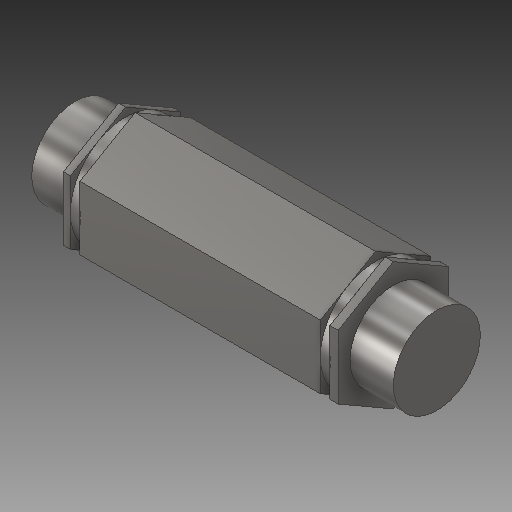
# Autodesk Inventor part: Hex Shaft 1
Saved by Autodesk Inventor 2019.4 (Build 234330000, 330)
## iProperties
Created: 2019-12-08
Part Number: Hex Shaft 1
Material: Steel, Mild
Document SubType Name: Modeling
Designer: admin
Density: 7.85 g/cm^3
Appearance: Semi-Polished
Mass: 40.5901 g
Surface Area: 20.2674 cm^2
Volume: 5.17072 cm^3
Author: admin
Autodesk Inventor part; units mm, degrees
ref_plane "YZ Plane" through (0, 0, 0) normal (1, 0, 0) x (0, 1, 0)
sketch "Sketch1" plane through (0, 0, 0) normal (0, 0, 1) x (1, 0, 0)
  line L0 (0, 0) -> (0, 5)
  line L1 (0, 5) -> (5, 5)
  line L2 (5, 5) -> (5, 8.4186)
  line L3 (5, 8.4186) -> (36.6, 8.4186)
  line L4 (36.6, 8.4186) -> (36.6, 5)
  line L5 (36.6, 5) -> (41.6, 5)
  line L6 (41.6, 5) -> (41.6, 0)
  line L7 (41.6, 0) -> (0, 0)
  dimension "d0" = 31.6
  dimension "d1" = 5
  dimension "d2" = 5
  dimension "d3" = 5
  constraints: 16 end point, 6 perpendicular, 2 point on line, 1 vertical
  measures "d0" distance of L2.end L3.end
  measures "d1" distance of L0.end L1.end
  measures "d2" distance of L4.end L5.end
  measures "d3" distance of L5.end L6.end
revolve "Revolution1" add sketch "Sketch1" angle 360 about axis through (41.6, 0, 0) along (-1, 0, 0)
sketch "Sketch2" plane through (36.6, 0, 0) normal (1, 0, 0) x (0, 0, -1)
  circle A0 centre (0, 0) radius 5 projected
  line L0 (0, 7.3323) -> (6.35, 3.6662)
  line L1 (6.35, 3.6662) -> (6.35, -3.6662)
  line L2 (6.35, -3.6662) -> (0, -7.3323)
  line L3 (0, -7.3323) -> (-6.35, -3.6662)
  line L4 (-6.35, -3.6662) -> (-6.35, 3.6662)
  line L5 (-6.35, 3.6662) -> (0, 7.3323)
  circle A1 centre (0, 0) radius 5 projected
  circle A2 centre (0, 0) radius 8.4186 projected
  dimension "d5" = 12.7
  constraints: 12 end point, 1 coincident, 13 other
  measures "d5" distance between parallel lines of L1 L4
extrude "Extrusion1" cut sketch "Sketch2" against normal up to surface (31.6 mm away) contours A2
ref_plane "Work Plane1" through (34.549, -3.6662, -6.35) normal (1, 0, 0) x (0, 0, -1)
sketch "Sketch3" plane through (34.549, -3.6662, -6.35) normal (1, 0, 0) x (0, 0, -1)
  circle A0 centre (-6.35, 3.6662) radius 5 projected
  circle A1 centre (-6.35, 3.6662) radius 6.35
  line L0 (0, 7.3323) -> (-6.35, 10.9985) projected
  circle A2 centre (-6.35, 3.6662) radius 5.85
  line L1 (-6.35, -3.6662) -> (0, 0) projected
  line L2 (0, 0) -> (0, 7.3323) projected
  line L3 (0, 7.3323) -> (-6.35, 10.9985) projected
  line L4 (-6.35, 10.9985) -> (-12.7, 7.3323) projected
  line L5 (-12.7, 7.3323) -> (-12.7, 0) projected
  line L6 (-12.7, 0) -> (-6.35, -3.6662) projected
  circle A3 centre (-6.35, 3.6662) radius 5 projected
  dimension "d9" = 0.5
  constraints: 2 centre point, 1 coincident, 1 tangent
  measures "d9" radial gap between concentric circles of A1 A2
extrude "Extrusion2" cut sketch "Sketch3" along normal blind 1.1 contours L2 L1 A1 | A1 L0 L2 | A1 L4 L0 | L1 L6 A1 | A1 L5 L4 | L6 L5 A1
ref_plane "Work Plane2" through (6.9, -3.6662, 6.35) normal (-1, 0, 0) x (0, 0, 1)
sketch "Sketch4" plane through (6.9, -3.6662, 6.35) normal (-1, 0, 0) x (0, 0, 1)
  line L0 (-12.7, 0) -> (-6.35, -3.6662) projected
  line L1 (-6.35, -3.6662) -> (0, 0) projected
  line L2 (0, 0) -> (0, 7.3323) projected
  line L3 (0, 7.3323) -> (-6.35, 10.9985) projected
  line L4 (-6.35, 10.9985) -> (-12.7, 7.3323) projected
  line L5 (-12.7, 7.3323) -> (-12.7, 0) projected
  circle A0 centre (-6.35, 3.6662) radius 5 projected
  circle A1 centre (-6.35, 3.6662) radius 5 projected
  circle A2 centre (-6.35, 3.6662) radius 6.35
  constraints: 1 centre point, 1 coincident
extrude "Extrusion3" cut sketch "Sketch4" along normal blind 1.1 contours L5 A2 L0 | A2 L1 L0 | L5 L4 A2 | A2 L2 L1 | L4 L3 A2 | A2 L3 L2
body "Solid1"
